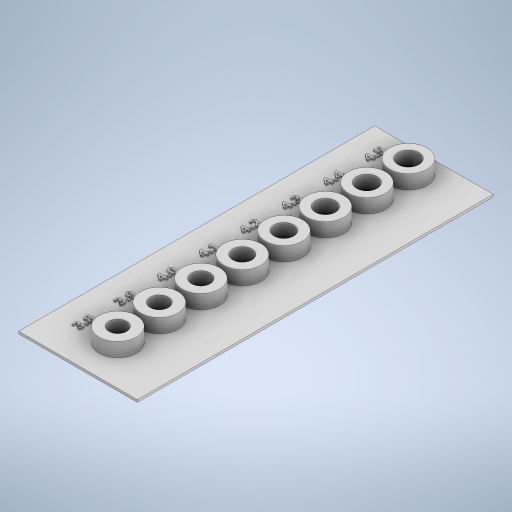
# Autodesk Inventor part: test plate press insert
Saved by Autodesk Inventor 2024.3 (Build 283343000, 343)
## iProperties
Created: 2024-05-10
Part Number: test plate press insert
Material: Generic
Document SubType Name: Modeling
Designer: atrus
Density: 1 g/cm^3
Appearance: Default
Author: atrus
Autodesk Inventor part; units mm, degrees
ref_plane "YZ Plane" through (0, 0, 0) normal (1, 0, 0) x (0, 1, 0)
ref_plane "XZ Plane" through (0, 0, 0) normal (0, 1, 0) x (-1, 0, 0)
ref_plane "XY Plane" through (0, 0, 0) normal (0, 0, 1) x (1, 0, 0)
sketch "Sketch1" plane through (0, 0, 0) normal (0, 1, 0) x (-1, 0, 0)
  line L0 (0, 0) -> (25.4, 0)
  line L1 (25.4, 0) -> (25.4, -76.2)
  line L2 (25.4, -76.2) -> (0, -76.2)
  line L3 (0, -76.2) -> (0, 0)
  dimension "d0" = 76.2
  dimension "d1" = 25.4
  constraints: 8 end point, 2 parallel, 1 horizontal, 1 perpendicular
  measures "d0" distance of L0.end L1.end
  measures "d1" distance of L1.end L2.end
extrude "Extrusion1" add sketch "Sketch1" along normal blind 0.5
sketch "Sketch2" plane through (0, 0.5, 0) normal (0, 1, 0) x (1, 0, 0)
  line L0 (-25.4, 0) -> (0, 0) projected
  line L1 (-12.7, 0) -> (-12.7, 76.2) construction
  line L2 (0, 76.2) -> (-25.4, 76.2) projected
  circle A0 centre (-12.7, 8.5029) radius 4
  circle A1 centre (-12.7, 17.3929) radius 4
  circle A2 centre (-12.7, 26.2829) radius 4
  circle A3 centre (-12.7, 35.1729) radius 4
  circle A4 centre (-12.7, 44.0629) radius 4
  circle A5 centre (-12.7, 52.9529) radius 4
  circle A6 centre (-12.7, 61.8429) radius 4
  circle A7 centre (-12.7, 70.7329) radius 4
  dimension "d4" = 8
  dimension "d7" = 8.89
  dimension "d22" = 8.89
  constraints: 8 centre point, 2 end point, 2 midpoint, 2 vertical, 1 point on line, 14 other
  measures "d4" diameter of A0
  measures "d7" distance of A0.centre A1.centre
  measures "d22" distance of A5.centre A6.centre
extrude "Extrusion2" add sketch "Sketch2" along normal blind 3
sketch "Sketch3" plane through (-12.7, 3.5, -8.5029) normal (0, 1, 0) x (1, 0, 0)
  circle A0 centre (0, 0) radius 4 construction
  circle A1 centre (0, 8.89) radius 4 construction
  circle A2 centre (0, 17.78) radius 4 construction
  circle A3 centre (0, 26.67) radius 4 construction
  circle A4 centre (0, 35.56) radius 4 construction
  circle A5 centre (0, 44.45) radius 4 construction
  circle A6 centre (0, 0) radius 1.9
  circle A7 centre (0, 8.89) radius 1.95
  circle A8 centre (0, 17.78) radius 2
  circle A9 centre (0, 26.67) radius 2.05
  circle A10 centre (0, 35.56) radius 2.1
  circle A11 centre (0, 44.45) radius 2.15
  circle A12 centre (0, 53.34) radius 4 construction
  circle A13 centre (0, 62.23) radius 4 construction
  circle A14 centre (0, 53.34) radius 2.2
  circle A15 centre (0, 62.23) radius 2.25
  line L0 (-12.7, -8.5029) -> (12.7, -8.5029) projected
  line L1 (0, 0) -> (-12.7, 0) construction
  line L2 (0, 8.89) -> (-12.7, 8.89) construction
  line L3 (0, 17.78) -> (-12.7, 17.78) construction
  line L4 (0, 26.67) -> (-12.7, 26.67) construction
  line L5 (0, 35.56) -> (-12.7, 35.56) construction
  line L6 (0, 44.45) -> (-12.7, 44.45) construction
  circle A16 centre (0, 53.34) radius 4 construction
  line L7 (0, 53.34) -> (-12.7, 53.34) construction
  line L8 (0, 62.23) -> (-12.7, 62.23) construction
  dimension "d14" = 3.8
  dimension "d15" = 3.9
  dimension "d16" = 4
  dimension "d17" = 4.1
  dimension "d18" = 4.2
  dimension "d19" = 4.3
  dimension "d27" = 4.4
  dimension "d28" = 4.5
  constraints: 16 end point, 8 centre point, 8 coincident
  measures "d14" diameter of A6
  measures "d15" diameter of A7
  measures "d16" diameter of A8
  measures "d17" diameter of A9
  measures "d18" diameter of A10
  measures "d19" diameter of A11
  measures "d27" diameter of A14
  measures "d28" diameter of A15
extrude "Extrusion3" cut sketch "Sketch3" against normal through all
sketch "Sketch4" plane through (0, 0.5, 0) normal (0, 1, 0) x (1, 0, 0)
  line L0 (-25.4, 0) -> (0, 0) construction
  line L1 (-25.4, 76.2) -> (-25.4, 0) construction
  circle A0 centre (-12.7, 8.5029) radius 1.9 construction
  line L2 (-12.7, 8.5029) -> (-25.4, 8.5029) construction
  line L3 (-12.7, 17.4678) -> (-25.4, 17.4678) construction
  circle A1 centre (-12.7, 26.2829) radius 2 construction
  circle A2 centre (-12.7, 35.1729) radius 2.05 construction
  circle A3 centre (-12.7, 44.0629) radius 2.1 construction
  circle A4 centre (-12.7, 52.9529) radius 2.15 construction
  circle A5 centre (-12.7, 61.8429) radius 2.2 construction
  circle A6 centre (-12.7, 70.7329) radius 2.25 construction
  line L4 (-12.7, 26.2829) -> (-25.4, 26.2829) construction
  line L5 (-12.7, 35.1729) -> (-25.4, 35.1729) construction
  line L6 (-12.7, 44.0629) -> (-25.4, 44.0629) construction
  line L7 (-12.7, 52.9529) -> (-25.4, 52.9529) construction
  line L8 (-12.7, 61.8429) -> (-25.4, 61.8429) construction
  line L9 (-12.7, 70.7329) -> (-25.4, 70.7329) construction
  line L10 (-19.05, 5.9382) -> (-19.05, 11.0677) construction
  line L11 (-19.05, 14.8282) -> (-19.05, 19.9577) construction
  line L12 (-19.05, 23.7182) -> (-19.05, 28.8477) construction
  line L13 (-19.05, 32.6082) -> (-19.05, 37.7377) construction
  line L14 (-19.05, 41.4982) -> (-19.05, 46.6277) construction
  line L15 (-19.05, 50.3882) -> (-19.05, 55.5177) construction
  line L16 (-19.05, 59.2782) -> (-19.05, 64.4077) construction
  line L17 (-19.05, 68.1682) -> (-19.05, 73.2977) construction
  spline S0 degree 2 poles (-19.5889, 8.0058) (-19.4578, 8.0058) (-19.2431, 7.9093) (-19.1681, 7.8157) knots 0 0 0 1 2 2 2
  spline S1 degree 2 poles (-19.1681, 7.8157) (-19.0932, 7.722) (-19.0125, 7.467) (-19.0125, 7.284) knots 0 0 0 1 2 2 2
  spline S2 degree 2 poles (-19.0125, 7.284) (-19.0125, 7.0765) (-19.0817, 6.7797) (-19.1249, 6.686) knots 0 0 0 1 2 2 2
  line L18 (-19.1249, 6.686) -> (-19.5111, 6.686)
  line L19 (-19.5111, 6.686) -> (-19.5111, 6.7293)
  spline S3 degree 2 poles (-19.5111, 6.7293) (-19.4491, 6.8272) (-19.3569, 7.0909) (-19.3569, 7.2004) knots 0 0 0 1 2 2 2
  spline S4 degree 2 poles (-19.3569, 7.2004) (-19.3569, 7.2653) (-19.38, 7.4165) (-19.4174, 7.4684) knots 0 0 0 1 2 2 2
  spline S5 degree 2 poles (-19.4174, 7.4684) (-19.4477, 7.5088) (-19.5356, 7.5577) (-19.6148, 7.5577) knots 0 0 0 1 2 2 2
  spline S6 degree 2 poles (-19.6148, 7.5577) (-19.6941, 7.5577) (-19.7791, 7.4886) (-19.7992, 7.431) knots 0 0 0 1 2 2 2
  spline S7 degree 2 poles (-19.7992, 7.431) (-19.8194, 7.3733) (-19.8237, 7.2134) (-19.8237, 7.1514) knots 0 0 0 1 2 2 2
  line L20 (-19.8237, 7.1514) -> (-19.8237, 7.0751)
  line L21 (-19.8237, 7.0751) -> (-20.1364, 7.0751)
  line L22 (-20.1364, 7.0751) -> (-20.1364, 7.1457)
  spline S8 degree 2 poles (-20.1364, 7.1457) (-20.1364, 7.2264) (-20.1508, 7.3632) (-20.1724, 7.4108) knots 0 0 0 1 2 2 2
  spline S9 degree 2 poles (-20.1724, 7.4108) (-20.1955, 7.4583) (-20.2762, 7.5116) (-20.3453, 7.5116) knots 0 0 0 1 2 2 2
  spline S10 degree 2 poles (-20.3453, 7.5116) (-20.4001, 7.5116) (-20.4678, 7.4612) (-20.4865, 7.4252) knots 0 0 0 1 2 2 2
  spline S11 degree 2 poles (-20.4865, 7.4252) (-20.5081, 7.382) (-20.5225, 7.2667) (-20.5225, 7.2264) knots 0 0 0 1 2 2 2
  spline S12 degree 2 poles (-20.5225, 7.2264) (-20.5225, 7.1615) (-20.4923, 7.0246) (-20.4678, 6.9612) knots 0 0 0 1 2 2 2
  spline S13 degree 2 poles (-20.4678, 6.9612) (-20.4491, 6.9108) (-20.3885, 6.8013) (-20.3727, 6.7754) knots 0 0 0 1 2 2 2
  line L23 (-20.3727, 6.7754) -> (-20.3727, 6.7379)
  line L24 (-20.3727, 6.7379) -> (-20.7531, 6.7379)
  spline S14 degree 2 poles (-20.7531, 6.7379) (-20.792, 6.8301) (-20.8655, 7.1413) (-20.8655, 7.3042) knots 0 0 0 1 2 2 2
  spline S15 degree 2 poles (-20.8655, 7.3042) (-20.8655, 7.4627) (-20.8107, 7.6961) (-20.7574, 7.7782) knots 0 0 0 1 2 2 2
  spline S16 degree 2 poles (-20.7574, 7.7782) (-20.7012, 7.869) (-20.5283, 7.9597) (-20.4202, 7.9597) knots 0 0 0 1 2 2 2
  spline S17 degree 2 poles (-20.4202, 7.9597) (-20.2675, 7.9597) (-20.0399, 7.784) (-20.0067, 7.6399) knots 0 0 0 1 2 2 2
  line L25 (-20.0067, 7.6399) -> (-19.9894, 7.6399)
  spline S18 degree 2 poles (-19.9894, 7.6399) (-19.9808, 7.7033) (-19.9347, 7.8243) (-19.8828, 7.8819) knots 0 0 0 1 2 2 2
  spline S19 degree 2 poles (-19.8828, 7.8819) (-19.8367, 7.9352) (-19.6897, 8.0058) (-19.5889, 8.0058) knots 0 0 0 1 2 2 2
  line L26 (-19.05, 8.7133) -> (-19.05, 8.2911)
  line L27 (-19.05, 8.2911) -> (-19.5197, 8.2911)
  line L28 (-19.5197, 8.2911) -> (-19.5197, 8.7133)
  line L29 (-19.5197, 8.7133) -> (-19.05, 8.7133)
  spline S20 degree 2 poles (-19.5442, 10.3674) (-19.4304, 10.3674) (-19.233, 10.2723) (-19.1609, 10.1815) knots 0 0 0 1 2 2 2
  spline S21 degree 2 poles (-19.1609, 10.1815) (-19.0889, 10.0907) (-19.0082, 9.83) (-19.0082, 9.6614) knots 0 0 0 1 2 2 2
  spline S22 degree 2 poles (-19.0082, 9.6614) (-19.0082, 9.4813) (-19.0903, 9.2118) (-19.1609, 9.1254) knots 0 0 0 1 2 2 2
  spline S23 degree 2 poles (-19.1609, 9.1254) (-19.2315, 9.0404) (-19.4232, 8.9597) (-19.5298, 8.9597) knots 0 0 0 1 2 2 2
  spline S24 degree 2 poles (-19.5298, 8.9597) (-19.6825, 8.9597) (-19.8857, 9.1283) (-19.9534, 9.2882) knots 0 0 0 1 2 2 2
  line L30 (-19.9534, 9.2882) -> (-19.9606, 9.2882)
  spline S25 degree 2 poles (-19.9606, 9.2882) (-20.037, 9.1311) (-20.2545, 9.0072) (-20.3885, 9.0072) knots 0 0 0 1 2 2 2
  spline S26 degree 2 poles (-20.3885, 9.0072) (-20.4865, 9.0072) (-20.658, 9.0937) (-20.7257, 9.1787) knots 0 0 0 1 2 2 2
  spline S27 degree 2 poles (-20.7257, 9.1787) (-20.7905, 9.2608) (-20.8683, 9.5101) (-20.8683, 9.6657) knots 0 0 0 1 2 2 2
  spline S28 degree 2 poles (-20.8683, 9.6657) (-20.8683, 9.83) (-20.7977, 10.0749) (-20.7401, 10.1541) knots 0 0 0 1 2 2 2
  spline S29 degree 2 poles (-20.7401, 10.1541) (-20.6825, 10.2348) (-20.5153, 10.3213) (-20.4188, 10.3213) knots 0 0 0 1 2 2 2
  spline S30 degree 2 poles (-20.4188, 10.3213) (-20.292, 10.3213) (-20.0888, 10.1743) (-20.0182, 10.023) knots 0 0 0 1 2 2 2
  line L31 (-20.0182, 10.023) -> (-20.0125, 10.023)
  spline S31 degree 2 poles (-20.0125, 10.023) (-19.9404, 10.2003) (-19.707, 10.3674) (-19.5442, 10.3674) knots 0 0 0 1 2 2 2
  spline S32 degree 2 poles (-19.5255, 9.9265) (-19.6134, 9.9265) (-19.7056, 9.8516) (-19.7647, 9.7305) knots 0 0 0 1 2 2 2
  spline S33 degree 2 poles (-19.7647, 9.7305) (-19.7805, 9.696) (-19.8309, 9.5648) (-19.8525, 9.5144) knots 0 0 0 1 2 2 2
  spline S34 degree 2 poles (-19.8525, 9.5144) (-19.8064, 9.4683) (-19.6681, 9.3948) (-19.586, 9.3948) knots 0 0 0 1 2 2 2
  spline S35 degree 2 poles (-19.586, 9.3948) (-19.4621, 9.3948) (-19.3137, 9.5533) (-19.3137, 9.6815) knots 0 0 0 1 2 2 2
  spline S36 degree 2 poles (-19.3137, 9.6815) (-19.3137, 9.7176) (-19.3367, 9.8069) (-19.3598, 9.8415) knots 0 0 0 1 2 2 2
  spline S37 degree 2 poles (-19.3598, 9.8415) (-19.3872, 9.8804) (-19.4621, 9.9265) (-19.5255, 9.9265) knots 0 0 0 1 2 2 2
  spline S38 degree 2 poles (-20.3669, 9.8876) (-20.4577, 9.8876) (-20.5658, 9.768) (-20.5658, 9.6657) knots 0 0 0 1 2 2 2
  spline S39 degree 2 poles (-20.5658, 9.6657) (-20.5658, 9.5677) (-20.4678, 9.4481) (-20.3957, 9.4481) knots 0 0 0 1 2 2 2
  spline S40 degree 2 poles (-20.3957, 9.4481) (-20.3251, 9.4481) (-20.2373, 9.5202) (-20.2012, 9.5965) knots 0 0 0 1 2 2 2
  spline S41 degree 2 poles (-20.2012, 9.5965) (-20.1839, 9.6297) (-20.1479, 9.7219) (-20.1191, 9.7983) knots 0 0 0 1 2 2 2
  spline S42 degree 2 poles (-20.1191, 9.7983) (-20.1796, 9.8444) (-20.2934, 9.8876) (-20.3669, 9.8876) knots 0 0 0 1 2 2 2
  spline S43 degree 2 poles (-19.5889, 16.8958) (-19.4578, 16.8958) (-19.2431, 16.7993) (-19.1681, 16.7057) knots 0 0 0 1 2 2 2
  spline S44 degree 2 poles (-19.1681, 16.7057) (-19.0932, 16.612) (-19.0125, 16.357) (-19.0125, 16.174) knots 0 0 0 1 2 2 2
  spline S45 degree 2 poles (-19.0125, 16.174) (-19.0125, 15.9665) (-19.0817, 15.6697) (-19.1249, 15.576) knots 0 0 0 1 2 2 2
  line L32 (-19.1249, 15.576) -> (-19.5111, 15.576)
  line L33 (-19.5111, 15.576) -> (-19.5111, 15.6193)
  spline S46 degree 2 poles (-19.5111, 15.6193) (-19.4491, 15.7172) (-19.3569, 15.9809) (-19.3569, 16.0904) knots 0 0 0 1 2 2 2
  spline S47 degree 2 poles (-19.3569, 16.0904) (-19.3569, 16.1553) (-19.38, 16.3065) (-19.4174, 16.3584) knots 0 0 0 1 2 2 2
  spline S48 degree 2 poles (-19.4174, 16.3584) (-19.4477, 16.3988) (-19.5356, 16.4477) (-19.6148, 16.4477) knots 0 0 0 1 2 2 2
  spline S49 degree 2 poles (-19.6148, 16.4477) (-19.6941, 16.4477) (-19.7791, 16.3786) (-19.7992, 16.321) knots 0 0 0 1 2 2 2
  spline S50 degree 2 poles (-19.7992, 16.321) (-19.8194, 16.2633) (-19.8237, 16.1034) (-19.8237, 16.0414) knots 0 0 0 1 2 2 2
  line L34 (-19.8237, 16.0414) -> (-19.8237, 15.9651)
  line L35 (-19.8237, 15.9651) -> (-20.1364, 15.9651)
  line L36 (-20.1364, 15.9651) -> (-20.1364, 16.0357)
  spline S51 degree 2 poles (-20.1364, 16.0357) (-20.1364, 16.1164) (-20.1508, 16.2532) (-20.1724, 16.3008) knots 0 0 0 1 2 2 2
  spline S52 degree 2 poles (-20.1724, 16.3008) (-20.1955, 16.3483) (-20.2762, 16.4016) (-20.3453, 16.4016) knots 0 0 0 1 2 2 2
  spline S53 degree 2 poles (-20.3453, 16.4016) (-20.4001, 16.4016) (-20.4678, 16.3512) (-20.4865, 16.3152) knots 0 0 0 1 2 2 2
  spline S54 degree 2 poles (-20.4865, 16.3152) (-20.5081, 16.272) (-20.5225, 16.1567) (-20.5225, 16.1164) knots 0 0 0 1 2 2 2
  spline S55 degree 2 poles (-20.5225, 16.1164) (-20.5225, 16.0515) (-20.4923, 15.9146) (-20.4678, 15.8512) knots 0 0 0 1 2 2 2
  spline S56 degree 2 poles (-20.4678, 15.8512) (-20.4491, 15.8008) (-20.3885, 15.6913) (-20.3727, 15.6654) knots 0 0 0 1 2 2 2
  line L37 (-20.3727, 15.6654) -> (-20.3727, 15.6279)
  line L38 (-20.3727, 15.6279) -> (-20.7531, 15.6279)
  spline S57 degree 2 poles (-20.7531, 15.6279) (-20.792, 15.7201) (-20.8655, 16.0313) (-20.8655, 16.1942) knots 0 0 0 1 2 2 2
  spline S58 degree 2 poles (-20.8655, 16.1942) (-20.8655, 16.3527) (-20.8107, 16.5861) (-20.7574, 16.6682) knots 0 0 0 1 2 2 2
  spline S59 degree 2 poles (-20.7574, 16.6682) (-20.7012, 16.759) (-20.5283, 16.8497) (-20.4202, 16.8497) knots 0 0 0 1 2 2 2
  spline S60 degree 2 poles (-20.4202, 16.8497) (-20.2675, 16.8497) (-20.0399, 16.674) (-20.0067, 16.5299) knots 0 0 0 1 2 2 2
  line L39 (-20.0067, 16.5299) -> (-19.9894, 16.5299)
  spline S61 degree 2 poles (-19.9894, 16.5299) (-19.9808, 16.5933) (-19.9347, 16.7143) (-19.8828, 16.7719) knots 0 0 0 1 2 2 2
  spline S62 degree 2 poles (-19.8828, 16.7719) (-19.8367, 16.8252) (-19.6897, 16.8958) (-19.5889, 16.8958) knots 0 0 0 1 2 2 2
  line L40 (-19.05, 17.6033) -> (-19.05, 17.1811)
  line L41 (-19.05, 17.1811) -> (-19.5197, 17.1811)
  line L42 (-19.5197, 17.1811) -> (-19.5197, 17.6033)
  line L43 (-19.5197, 17.6033) -> (-19.05, 17.6033)
  spline S63 degree 2 poles (-20.0384, 19.2156) (-19.8122, 19.2156) (-19.4347, 19.1104) (-19.2993, 18.9995) knots 0 0 0 1 2 2 2
  spline S64 degree 2 poles (-19.2993, 18.9995) (-19.1624, 18.8842) (-19.0154, 18.5442) (-19.0154, 18.2963) knots 0 0 0 1 2 2 2
  spline S65 degree 2 poles (-19.0154, 18.2963) (-19.0154, 18.2128) (-19.037, 18.0312) (-19.0457, 18.001) knots 0 0 0 1 2 2 2
  line L44 (-19.0457, 18.001) -> (-19.3944, 18.001)
  line L45 (-19.3944, 18.001) -> (-19.3944, 18.0356)
  spline S66 degree 2 poles (-19.3944, 18.0356) (-19.3771, 18.0687) (-19.3396, 18.1926) (-19.3396, 18.3007) knots 0 0 0 1 2 2 2
  spline S67 degree 2 poles (-19.3396, 18.3007) (-19.3396, 18.3886) (-19.3857, 18.5514) (-19.4361, 18.609) knots 0 0 0 1 2 2 2
  spline S68 degree 2 poles (-19.4361, 18.609) (-19.4895, 18.671) (-19.6465, 18.7517) (-19.7647, 18.7661) knots 0 0 0 1 2 2 2
  spline S69 degree 2 poles (-19.7647, 18.7661) (-19.7056, 18.671) (-19.6422, 18.5067) (-19.6422, 18.3842) knots 0 0 0 1 2 2 2
  spline S70 degree 2 poles (-19.6422, 18.3842) (-19.6422, 18.2935) (-19.6912, 18.1249) (-19.743, 18.0557) knots 0 0 0 1 2 2 2
  spline S71 degree 2 poles (-19.743, 18.0557) (-19.8136, 17.9635) (-20.0399, 17.8554) (-20.2185, 17.8554) knots 0 0 0 1 2 2 2
  spline S72 degree 2 poles (-20.2185, 17.8554) (-20.3583, 17.8554) (-20.5931, 17.9505) (-20.6796, 18.037) knots 0 0 0 1 2 2 2
  spline S73 degree 2 poles (-20.6796, 18.037) (-20.766, 18.1234) (-20.864, 18.3742) (-20.864, 18.5283) knots 0 0 0 1 2 2 2
  spline S74 degree 2 poles (-20.864, 18.5283) (-20.864, 18.6839) (-20.7776, 18.9246) (-20.6868, 19.011) knots 0 0 0 1 2 2 2
  spline S75 degree 2 poles (-20.6868, 19.011) (-20.5859, 19.1119) (-20.2661, 19.2156) (-20.0384, 19.2156) knots 0 0 0 1 2 2 2
  spline S76 degree 2 poles (-20.1047, 18.7733) (-20.2502, 18.7733) (-20.4375, 18.7243) (-20.4894, 18.6796) knots 0 0 0 1 2 2 2
  spline S77 degree 2 poles (-20.4894, 18.6796) (-20.5283, 18.6494) (-20.5614, 18.5715) (-20.5614, 18.5269) knots 0 0 0 1 2 2 2
  spline S78 degree 2 poles (-20.5614, 18.5269) (-20.5614, 18.4865) (-20.5297, 18.4116) (-20.4894, 18.377) knots 0 0 0 1 2 2 2
  spline S79 degree 2 poles (-20.4894, 18.377) (-20.4548, 18.3468) (-20.3208, 18.3036) (-20.2416, 18.3036) knots 0 0 0 1 2 2 2
  spline S80 degree 2 poles (-20.2416, 18.3036) (-20.1551, 18.3036) (-20.0442, 18.3482) (-20.011, 18.3857) knots 0 0 0 1 2 2 2
  spline S81 degree 2 poles (-20.011, 18.3857) (-19.9779, 18.4246) (-19.952, 18.5211) (-19.952, 18.5816) knots 0 0 0 1 2 2 2
  spline S82 degree 2 poles (-19.952, 18.5816) (-19.952, 18.6321) (-19.9793, 18.7372) (-19.9938, 18.7704) knots 0 0 0 1 2 2 2
  spline S83 degree 2 poles (-19.9938, 18.7704) (-20.0067, 18.7704) (-20.0557, 18.7733) (-20.1047, 18.7733) knots 0 0 0 1 2 2 2
  line L46 (-19.465, 25.8521) -> (-19.465, 25.6115)
  line L47 (-19.465, 25.6115) -> (-19.0457, 25.6115)
  line L48 (-19.0457, 25.6115) -> (-19.0457, 25.1807)
  line L49 (-19.0457, 25.1807) -> (-19.465, 25.1807)
  line L50 (-19.465, 25.1807) -> (-19.465, 24.3969)
  line L51 (-19.465, 24.3969) -> (-19.7964, 24.3969)
  line L52 (-19.7964, 24.3969) -> (-20.828, 25.1663)
  line L53 (-20.828, 25.1663) -> (-20.828, 25.6115)
  line L54 (-20.828, 25.6115) -> (-19.7848, 25.6115)
  line L55 (-19.7848, 25.6115) -> (-19.7848, 25.8521)
  line L56 (-19.7848, 25.8521) -> (-19.465, 25.8521)
  line L57 (-19.7848, 25.1807) -> (-20.39, 25.1807)
  line L58 (-20.39, 25.1807) -> (-19.7848, 24.7297)
  line L59 (-19.7848, 24.7297) -> (-19.7848, 25.1807)
  line L60 (-19.05, 26.4933) -> (-19.05, 26.0711)
  line L61 (-19.05, 26.0711) -> (-19.5197, 26.0711)
  line L62 (-19.5197, 26.0711) -> (-19.5197, 26.4933)
  line L63 (-19.5197, 26.4933) -> (-19.05, 26.4933)
  spline S84 degree 2 poles (-19.939, 28.1287) (-19.7085, 28.1287) (-19.3627, 28.0552) (-19.246, 27.973) knots 0 0 0 1 2 2 2
  spline S85 degree 2 poles (-19.246, 27.973) (-19.1307, 27.8924) (-19.0125, 27.6316) (-19.0125, 27.4443) knots 0 0 0 1 2 2 2
  spline S86 degree 2 poles (-19.0125, 27.4443) (-19.0125, 27.2555) (-19.1307, 26.9962) (-19.2488, 26.914) knots 0 0 0 1 2 2 2
  spline S87 degree 2 poles (-19.2488, 26.914) (-19.3655, 26.8319) (-19.7085, 26.7584) (-19.939, 26.7584) knots 0 0 0 1 2 2 2
  spline S88 degree 2 poles (-19.939, 26.7584) (-20.1753, 26.7584) (-20.5096, 26.8319) (-20.6306, 26.9155) knots 0 0 0 1 2 2 2
  spline S89 degree 2 poles (-20.6306, 26.9155) (-20.7488, 26.999) (-20.864, 27.2627) (-20.864, 27.4443) knots 0 0 0 1 2 2 2
  spline S90 degree 2 poles (-20.864, 27.4443) (-20.864, 27.6359) (-20.743, 27.8924) (-20.6234, 27.9745) knots 0 0 0 1 2 2 2
  spline S91 degree 2 poles (-20.6234, 27.9745) (-20.5067, 28.0552) (-20.1623, 28.1287) (-19.939, 28.1287) knots 0 0 0 1 2 2 2
  spline S92 degree 2 poles (-19.939, 27.6806) (-20.269, 27.6806) (-20.5355, 27.5725) (-20.5355, 27.4443) knots 0 0 0 1 2 2 2
  spline S93 degree 2 poles (-20.5355, 27.4443) (-20.5355, 27.316) (-20.269, 27.2065) (-19.9376, 27.2065) knots 0 0 0 1 2 2 2
  spline S94 degree 2 poles (-19.9376, 27.2065) (-19.6119, 27.2065) (-19.3411, 27.316) (-19.3411, 27.4443) knots 0 0 0 1 2 2 2
  spline S95 degree 2 poles (-19.3411, 27.4443) (-19.3411, 27.5711) (-19.6119, 27.6806) (-19.939, 27.6806) knots 0 0 0 1 2 2 2
  line L64 (-19.465, 34.7421) -> (-19.465, 34.5015)
  line L65 (-19.465, 34.5015) -> (-19.0457, 34.5015)
  line L66 (-19.0457, 34.5015) -> (-19.0457, 34.0707)
  line L67 (-19.0457, 34.0707) -> (-19.465, 34.0707)
  line L68 (-19.465, 34.0707) -> (-19.465, 33.2869)
  line L69 (-19.465, 33.2869) -> (-19.7964, 33.2869)
  line L70 (-19.7964, 33.2869) -> (-20.828, 34.0563)
  line L71 (-20.828, 34.0563) -> (-20.828, 34.5015)
  line L72 (-20.828, 34.5015) -> (-19.7848, 34.5015)
  line L73 (-19.7848, 34.5015) -> (-19.7848, 34.7421)
  line L74 (-19.7848, 34.7421) -> (-19.465, 34.7421)
  line L75 (-19.7848, 34.0707) -> (-20.39, 34.0707)
  line L76 (-20.39, 34.0707) -> (-19.7848, 33.6197)
  line L77 (-19.7848, 33.6197) -> (-19.7848, 34.0707)
  line L78 (-19.05, 35.3833) -> (-19.05, 34.9611)
  line L79 (-19.05, 34.9611) -> (-19.5197, 34.9611)
  line L80 (-19.5197, 34.9611) -> (-19.5197, 35.3833)
  line L81 (-19.5197, 35.3833) -> (-19.05, 35.3833)
  line L82 (-19.05, 36.9625) -> (-19.05, 35.7882)
  line L83 (-19.05, 35.7882) -> (-19.3598, 35.7882)
  line L84 (-19.3598, 35.7882) -> (-19.3598, 36.1628)
  line L85 (-19.3598, 36.1628) -> (-20.3007, 36.1628)
  line L86 (-20.3007, 36.1628) -> (-20.3007, 35.7882)
  line L87 (-20.3007, 35.7882) -> (-20.5903, 35.7882)
  spline S96 degree 2 poles (-20.5903, 35.7882) (-20.5903, 35.8703) (-20.6119, 36.0331) (-20.6349, 36.0821) knots 0 0 0 1 2 2 2
  spline S97 degree 2 poles (-20.6349, 36.0821) (-20.6637, 36.1383) (-20.7603, 36.2017) (-20.8323, 36.2075) knots 0 0 0 1 2 2 2
  line L88 (-20.8323, 36.2075) -> (-20.8323, 36.5965)
  line L89 (-20.8323, 36.5965) -> (-19.3598, 36.5965)
  line L90 (-19.3598, 36.5965) -> (-19.3598, 36.9625)
  line L91 (-19.3598, 36.9625) -> (-19.05, 36.9625)
  line L92 (-19.465, 43.6321) -> (-19.465, 43.3915)
  line L93 (-19.465, 43.3915) -> (-19.0457, 43.3915)
  line L94 (-19.0457, 43.3915) -> (-19.0457, 42.9607)
  line L95 (-19.0457, 42.9607) -> (-19.465, 42.9607)
  line L96 (-19.465, 42.9607) -> (-19.465, 42.1769)
  line L97 (-19.465, 42.1769) -> (-19.7964, 42.1769)
  line L98 (-19.7964, 42.1769) -> (-20.828, 42.9463)
  line L99 (-20.828, 42.9463) -> (-20.828, 43.3915)
  line L100 (-20.828, 43.3915) -> (-19.7848, 43.3915)
  line L101 (-19.7848, 43.3915) -> (-19.7848, 43.6321)
  line L102 (-19.7848, 43.6321) -> (-19.465, 43.6321)
  line L103 (-19.7848, 42.9607) -> (-20.39, 42.9607)
  line L104 (-20.39, 42.9607) -> (-19.7848, 42.5097)
  line L105 (-19.7848, 42.5097) -> (-19.7848, 42.9607)
  line L106 (-19.05, 44.2733) -> (-19.05, 43.8511)
  line L107 (-19.05, 43.8511) -> (-19.5197, 43.8511)
  line L108 (-19.5197, 43.8511) -> (-19.5197, 44.2733)
  line L109 (-19.5197, 44.2733) -> (-19.05, 44.2733)
  line L110 (-19.05, 45.9317) -> (-19.05, 44.6249)
  line L111 (-19.05, 44.6249) -> (-19.3396, 44.6249)
  spline S98 degree 2 poles (-19.3396, 44.6249) (-19.4722, 44.7906) (-19.7056, 45.0557) (-19.8108, 45.1551) knots 0 0 0 1 2 2 2
  spline S99 degree 2 poles (-19.8108, 45.1551) (-19.9476, 45.2862) (-20.1566, 45.4029) (-20.2661, 45.4029) knots 0 0 0 1 2 2 2
  spline S100 degree 2 poles (-20.2661, 45.4029) (-20.39, 45.4029) (-20.5225, 45.2545) (-20.5225, 45.122) knots 0 0 0 1 2 2 2
  spline S101 degree 2 poles (-20.5225, 45.122) (-20.5225, 45.0542) (-20.4894, 44.9332) (-20.4635, 44.8713) knots 0 0 0 1 2 2 2
  spline S102 degree 2 poles (-20.4635, 44.8713) (-20.4361, 44.8107) (-20.3785, 44.7243) (-20.364, 44.7027) knots 0 0 0 1 2 2 2
  line L112 (-20.364, 44.7027) -> (-20.364, 44.6681)
  line L113 (-20.364, 44.6681) -> (-20.7516, 44.6681)
  spline S103 degree 2 poles (-20.7516, 44.6681) (-20.7877, 44.743) (-20.8626, 45.0629) (-20.8626, 45.2113) knots 0 0 0 1 2 2 2
  spline S104 degree 2 poles (-20.8626, 45.2113) (-20.8626, 45.5283) (-20.5802, 45.8539) (-20.3251, 45.8539) knots 0 0 0 1 2 2 2
  spline S105 degree 2 poles (-20.3251, 45.8539) (-20.1681, 45.8539) (-19.8655, 45.7055) (-19.6926, 45.534) knots 0 0 0 1 2 2 2
  spline S106 degree 2 poles (-19.6926, 45.534) (-19.586, 45.426) (-19.4203, 45.2228) (-19.3857, 45.1782) knots 0 0 0 1 2 2 2
  line L114 (-19.3857, 45.1782) -> (-19.3857, 45.9317)
  line L115 (-19.3857, 45.9317) -> (-19.05, 45.9317)
  line L116 (-19.465, 52.5221) -> (-19.465, 52.2815)
  line L117 (-19.465, 52.2815) -> (-19.0457, 52.2815)
  line L118 (-19.0457, 52.2815) -> (-19.0457, 51.8507)
  line L119 (-19.0457, 51.8507) -> (-19.465, 51.8507)
  line L120 (-19.465, 51.8507) -> (-19.465, 51.0669)
  line L121 (-19.465, 51.0669) -> (-19.7964, 51.0669)
  line L122 (-19.7964, 51.0669) -> (-20.828, 51.8363)
  line L123 (-20.828, 51.8363) -> (-20.828, 52.2815)
  line L124 (-20.828, 52.2815) -> (-19.7848, 52.2815)
  line L125 (-19.7848, 52.2815) -> (-19.7848, 52.5221)
  line L126 (-19.7848, 52.5221) -> (-19.465, 52.5221)
  line L127 (-19.7848, 51.8507) -> (-20.39, 51.8507)
  line L128 (-20.39, 51.8507) -> (-19.7848, 51.3997)
  line L129 (-19.7848, 51.3997) -> (-19.7848, 51.8507)
  line L130 (-19.05, 53.1633) -> (-19.05, 52.7411)
  line L131 (-19.05, 52.7411) -> (-19.5197, 52.7411)
  line L132 (-19.5197, 52.7411) -> (-19.5197, 53.1633)
  line L133 (-19.5197, 53.1633) -> (-19.05, 53.1633)
  spline S107 degree 2 poles (-19.5889, 54.777) (-19.4578, 54.777) (-19.2431, 54.6805) (-19.1681, 54.5869) knots 0 0 0 1 2 2 2
  spline S108 degree 2 poles (-19.1681, 54.5869) (-19.0932, 54.4932) (-19.0125, 54.2382) (-19.0125, 54.0552) knots 0 0 0 1 2 2 2
  spline S109 degree 2 poles (-19.0125, 54.0552) (-19.0125, 53.8477) (-19.0817, 53.5509) (-19.1249, 53.4572) knots 0 0 0 1 2 2 2
  line L134 (-19.1249, 53.4572) -> (-19.5111, 53.4572)
  line L135 (-19.5111, 53.4572) -> (-19.5111, 53.5005)
  spline S110 degree 2 poles (-19.5111, 53.5005) (-19.4491, 53.5984) (-19.3569, 53.8621) (-19.3569, 53.9716) knots 0 0 0 1 2 2 2
  spline S111 degree 2 poles (-19.3569, 53.9716) (-19.3569, 54.0365) (-19.38, 54.1877) (-19.4174, 54.2396) knots 0 0 0 1 2 2 2
  spline S112 degree 2 poles (-19.4174, 54.2396) (-19.4477, 54.28) (-19.5356, 54.3289) (-19.6148, 54.3289) knots 0 0 0 1 2 2 2
  spline S113 degree 2 poles (-19.6148, 54.3289) (-19.6941, 54.3289) (-19.7791, 54.2598) (-19.7992, 54.2021) knots 0 0 0 1 2 2 2
  spline S114 degree 2 poles (-19.7992, 54.2021) (-19.8194, 54.1445) (-19.8237, 53.9846) (-19.8237, 53.9226) knots 0 0 0 1 2 2 2
  line L136 (-19.8237, 53.9226) -> (-19.8237, 53.8463)
  line L137 (-19.8237, 53.8463) -> (-20.1364, 53.8463)
  line L138 (-20.1364, 53.8463) -> (-20.1364, 53.9169)
  spline S115 degree 2 poles (-20.1364, 53.9169) (-20.1364, 53.9975) (-20.1508, 54.1344) (-20.1724, 54.182) knots 0 0 0 1 2 2 2
  spline S116 degree 2 poles (-20.1724, 54.182) (-20.1955, 54.2295) (-20.2762, 54.2828) (-20.3453, 54.2828) knots 0 0 0 1 2 2 2
  spline S117 degree 2 poles (-20.3453, 54.2828) (-20.4001, 54.2828) (-20.4678, 54.2324) (-20.4865, 54.1964) knots 0 0 0 1 2 2 2
  spline S118 degree 2 poles (-20.4865, 54.1964) (-20.5081, 54.1532) (-20.5225, 54.0379) (-20.5225, 53.9975) knots 0 0 0 1 2 2 2
  spline S119 degree 2 poles (-20.5225, 53.9975) (-20.5225, 53.9327) (-20.4923, 53.7958) (-20.4678, 53.7324) knots 0 0 0 1 2 2 2
  spline S120 degree 2 poles (-20.4678, 53.7324) (-20.4491, 53.682) (-20.3885, 53.5725) (-20.3727, 53.5466) knots 0 0 0 1 2 2 2
  line L139 (-20.3727, 53.5466) -> (-20.3727, 53.5091)
  line L140 (-20.3727, 53.5091) -> (-20.7531, 53.5091)
  spline S121 degree 2 poles (-20.7531, 53.5091) (-20.792, 53.6013) (-20.8655, 53.9125) (-20.8655, 54.0754) knots 0 0 0 1 2 2 2
  spline S122 degree 2 poles (-20.8655, 54.0754) (-20.8655, 54.2338) (-20.8107, 54.4673) (-20.7574, 54.5494) knots 0 0 0 1 2 2 2
  spline S123 degree 2 poles (-20.7574, 54.5494) (-20.7012, 54.6402) (-20.5283, 54.7309) (-20.4202, 54.7309) knots 0 0 0 1 2 2 2
  spline S124 degree 2 poles (-20.4202, 54.7309) (-20.2675, 54.7309) (-20.0399, 54.5552) (-20.0067, 54.4111) knots 0 0 0 1 2 2 2
  line L141 (-20.0067, 54.4111) -> (-19.9894, 54.4111)
  spline S125 degree 2 poles (-19.9894, 54.4111) (-19.9808, 54.4745) (-19.9347, 54.5955) (-19.8828, 54.6531) knots 0 0 0 1 2 2 2
  spline S126 degree 2 poles (-19.8828, 54.6531) (-19.8367, 54.7064) (-19.6897, 54.777) (-19.5889, 54.777) knots 0 0 0 1 2 2 2
  line L142 (-19.465, 61.4121) -> (-19.465, 61.1715)
  line L143 (-19.465, 61.1715) -> (-19.0457, 61.1715)
  line L144 (-19.0457, 61.1715) -> (-19.0457, 60.7407)
  line L145 (-19.0457, 60.7407) -> (-19.465, 60.7407)
  line L146 (-19.465, 60.7407) -> (-19.465, 59.9569)
  line L147 (-19.465, 59.9569) -> (-19.7964, 59.9569)
  line L148 (-19.7964, 59.9569) -> (-20.828, 60.7263)
  line L149 (-20.828, 60.7263) -> (-20.828, 61.1715)
  line L150 (-20.828, 61.1715) -> (-19.7848, 61.1715)
  line L151 (-19.7848, 61.1715) -> (-19.7848, 61.4121)
  line L152 (-19.7848, 61.4121) -> (-19.465, 61.4121)
  line L153 (-19.7848, 60.7407) -> (-20.39, 60.7407)
  line L154 (-20.39, 60.7407) -> (-19.7848, 60.2897)
  line L155 (-19.7848, 60.2897) -> (-19.7848, 60.7407)
  line L156 (-19.05, 62.0533) -> (-19.05, 61.6311)
  line L157 (-19.05, 61.6311) -> (-19.5197, 61.6311)
  line L158 (-19.5197, 61.6311) -> (-19.5197, 62.0533)
  line L159 (-19.5197, 62.0533) -> (-19.05, 62.0533)
  line L160 (-19.465, 63.7333) -> (-19.465, 63.4927)
  line L161 (-19.465, 63.4927) -> (-19.0457, 63.4927)
  line L162 (-19.0457, 63.4927) -> (-19.0457, 63.0619)
  line L163 (-19.0457, 63.0619) -> (-19.465, 63.0619)
  line L164 (-19.465, 63.0619) -> (-19.465, 62.2781)
  line L165 (-19.465, 62.2781) -> (-19.7964, 62.2781)
  line L166 (-19.7964, 62.2781) -> (-20.828, 63.0475)
  line L167 (-20.828, 63.0475) -> (-20.828, 63.4927)
  line L168 (-20.828, 63.4927) -> (-19.7848, 63.4927)
  line L169 (-19.7848, 63.4927) -> (-19.7848, 63.7333)
  line L170 (-19.7848, 63.7333) -> (-19.465, 63.7333)
  line L171 (-19.7848, 63.0619) -> (-20.39, 63.0619)
  line L172 (-20.39, 63.0619) -> (-19.7848, 62.6109)
  line L173 (-19.7848, 62.6109) -> (-19.7848, 63.0619)
  line L174 (-19.465, 70.3021) -> (-19.465, 70.0615)
  line L175 (-19.465, 70.0615) -> (-19.0457, 70.0615)
  line L176 (-19.0457, 70.0615) -> (-19.0457, 69.6307)
  line L177 (-19.0457, 69.6307) -> (-19.465, 69.6307)
  line L178 (-19.465, 69.6307) -> (-19.465, 68.8469)
  line L179 (-19.465, 68.8469) -> (-19.7964, 68.8469)
  line L180 (-19.7964, 68.8469) -> (-20.828, 69.6163)
  line L181 (-20.828, 69.6163) -> (-20.828, 70.0615)
  line L182 (-20.828, 70.0615) -> (-19.7848, 70.0615)
  line L183 (-19.7848, 70.0615) -> (-19.7848, 70.3021)
  line L184 (-19.7848, 70.3021) -> (-19.465, 70.3021)
  line L185 (-19.7848, 69.6307) -> (-20.39, 69.6307)
  line L186 (-20.39, 69.6307) -> (-19.7848, 69.1797)
  line L187 (-19.7848, 69.1797) -> (-19.7848, 69.6307)
  line L188 (-19.05, 70.9433) -> (-19.05, 70.5211)
  line L189 (-19.05, 70.5211) -> (-19.5197, 70.5211)
  line L190 (-19.5197, 70.5211) -> (-19.5197, 70.9433)
  line L191 (-19.5197, 70.9433) -> (-19.05, 70.9433)
  spline S127 degree 2 poles (-19.6523, 72.5614) (-19.5125, 72.5614) (-19.2762, 72.4663) (-19.1912, 72.3726) knots 0 0 0 1 2 2 2
  spline S128 degree 2 poles (-19.1912, 72.3726) (-19.1062, 72.279) (-19.0125, 72.0225) (-19.0125, 71.8352) knots 0 0 0 1 2 2 2
  spline S129 degree 2 poles (-19.0125, 71.8352) (-19.014, 71.6363) (-19.0788, 71.3511) (-19.1206, 71.2574) knots 0 0 0 1 2 2 2
  line L192 (-19.1206, 71.2574) -> (-19.5082, 71.2574)
  line L193 (-19.5082, 71.2574) -> (-19.5082, 71.2977)
  spline S130 degree 2 poles (-19.5082, 71.2977) (-19.4895, 71.3323) (-19.4405, 71.4159) (-19.4145, 71.4836) knots 0 0 0 1 2 2 2
  spline S131 degree 2 poles (-19.4145, 71.4836) (-19.39, 71.547) (-19.3569, 71.6781) (-19.3569, 71.7574) knots 0 0 0 1 2 2 2
  spline S132 degree 2 poles (-19.3569, 71.7574) (-19.3569, 71.8265) (-19.3915, 71.9879) (-19.4376, 72.0369) knots 0 0 0 1 2 2 2
  spline S133 degree 2 poles (-19.4376, 72.0369) (-19.4736, 72.0729) (-19.5615, 72.1133) (-19.635, 72.1133) knots 0 0 0 1 2 2 2
  spline S134 degree 2 poles (-19.635, 72.1133) (-19.6984, 72.1133) (-19.7877, 72.0614) (-19.8151, 72.0196) knots 0 0 0 1 2 2 2
  spline S135 degree 2 poles (-19.8151, 72.0196) (-19.8554, 71.9591) (-19.8785, 71.7862) (-19.8785, 71.7242) knots 0 0 0 1 2 2 2
  spline S136 degree 2 poles (-19.8785, 71.7242) (-19.8785, 71.6263) (-19.8468, 71.4404) (-19.8295, 71.3727) knots 0 0 0 1 2 2 2
  line L194 (-19.8295, 71.3727) -> (-19.8295, 71.3338)
  line L195 (-19.8295, 71.3338) -> (-20.828, 71.3338)
  line L196 (-20.828, 71.3338) -> (-20.828, 72.5124)
  line L197 (-20.828, 72.5124) -> (-20.4923, 72.5124)
  line L198 (-20.4923, 72.5124) -> (-20.4923, 71.7559)
  line L199 (-20.4923, 71.7559) -> (-20.1969, 71.7559)
  spline S137 degree 2 poles (-20.1969, 71.7559) (-20.1998, 71.792) (-20.2027, 71.8914) (-20.2027, 71.9188) knots 0 0 0 1 2 2 2
  spline S138 degree 2 poles (-20.2027, 71.9188) (-20.2027, 72.047) (-20.1508, 72.2631) (-20.0975, 72.3481) knots 0 0 0 1 2 2 2
  spline S139 degree 2 poles (-20.0975, 72.3481) (-20.0312, 72.449) (-19.8108, 72.5614) (-19.6523, 72.5614) knots 0 0 0 1 2 2 2
  point P0 (-19.05, 8.5029)
  point P1 (-19.05, 17.3929)
  point P2 (-19.05, 26.2829)
  point P3 (-19.05, 35.1729)
  point P4 (-19.05, 44.0629)
  point P5 (-19.05, 52.9529)
  point P6 (-19.05, 61.8429)
  point P7 (-19.05, 70.7329)
  dimension "d33" = 6.35
  dimension "d36" = 8.89
  constraints: 32 end point, 10 vertical, 8 horizontal, 2 midpoint, 1 collinear, 36 other
  measures "d36" distance of L10.start L11.start
extrude "Extrusion4" add sketch "Sketch4" along normal blind 0.3
body "Solid1"
